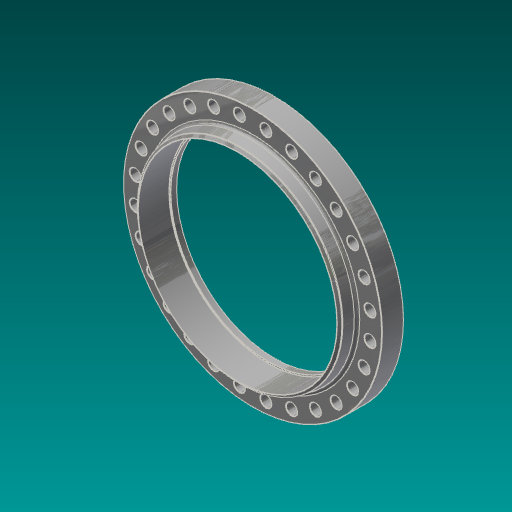
# Autodesk Inventor part: A1-19027-200-03 30in CL300 flange
Saved by Autodesk Inventor 2017.3 (Build 213257000, 257)
## iProperties
Created: 2019-06-26
Part Number: A1-19027-200-03 30in CL300 flange
Material: Steel, Mild
Document SubType Name: Modeling
Designer: Graeme_Van_Dongen
Density: 7.85 g/cm^3
Appearance: Steel
Mass: 267042 g
Surface Area: 19229.6 cm^2
Volume: 34018.1 cm^3
Description: 30" CLASS 300 FFWN FLANGE, A350 LF2, Ø32 1/2" BORE
Author: Graeme_Van_Dongen
Autodesk Inventor part; units mm, degrees
ref_plane "YZ Plane" through (0, 0, 0) normal (1, 0, 0) x (0, 1, 0)
ref_plane "XZ Plane" through (0, 0, 0) normal (0, 1, 0) x (-1, 0, 0)
sketch "Sketch1" plane through (0, 0, 0) normal (0, 0, 1) x (1, 0, 0)
  circle A0 centre (0, 0) radius 546.1
  dimension "d0" = 1092.2
  constraints: 1 centre point, 1 coincident
  measures "d0" diameter of A0
extrude "Extrusion1" add sketch "Sketch1" along normal blind 92.075
sketch "Sketch2" plane through (0, 0, 92.075) normal (0, 0, 1) x (1, 0, 0)
  line L0 (-55.8115, -495.3407) -> (55.8115, 495.3407) construction
  line L1 (0, -764.54) -> (0, 764.54) construction
  point P0 (0, 0)
  point P1 (0, 0)
  dimension "d3" = 996.95
  dimension "d4" = 6.429
  constraints: 2 coincident, 2 end point, 1 midpoint
  measures "d3" distance of L0.start L0.end
  measures "d4" angle of L0 L1
hole "Hole1" at (55.8115, 495.3407, 92.075) direction (0, 0, -1) diameter 47.625 end through all
chamfer "Chamfer1" distance 1.5875 angle 45 2 edges at (55.8115, 519.1532, 92.075) (55.8115, 519.1532, 0)
pattern_circular "Circular Pattern1" count 28 over 360 about axis through (0, 0, -10) along (0, 0, 1) of "Hole1", "Chamfer1"
chamfer "Chamfer2" distance 1.5875 angle 45 2 edges at (-546.1, 0, 92.075) (-546.1, 0, 0)
sketch "Sketch3" plane through (0, 0, 92.075) normal (0, 0, 1) x (1, 0, 0)
  circle A0 centre (0, 0) radius 441.325
  dimension "d21" = 882.65
  constraints: 1 centre point, 1 coincident
  measures "d21" diameter of A0
ref_plane "Work Plane1" through (0, 0, 155.575) normal (0, 0, 1) x (1, 0, 0)
sketch "Sketch4" plane through (0, 0, 155.575) normal (0, 0, 1) x (1, 0, 0)
  circle A0 centre (0, 0) radius 431.8
  dimension "d23" = 863.6
  constraints: 1 centre point, 1 coincident
  measures "d23" diameter of A0
extrude "Extrusion2" add sketch "Sketch4" against normal blind 12.7
loft "Loft1" add profiles "Sketch3" section 1 edges at (-431.8, 0, 142.875)
fillet "Fillet1" radius 12.7 1 edges at (-441.325, 0, 92.075)
sketch "Sketch5" plane through (0, 0, 0) normal (1, 0, 0) x (0, 1, 0)
  line L0 (439.3826, 102.4345) -> (431.8, 142.875) projected
  arc A0 (439.3826, 102.4345) -> (451.8651, 92.075) centre (451.8651, 104.775) ccw projected
  line L1 (431.8, 155.575) -> (431.8, 142.875) construction
  line L2 (0, -30.7975) -> (0, 184.785) projected
  line L3 (0, 0) -> (419.1, 0)
  line L4 (419.1, 0) -> (419.1, 155.575)
  line L5 (420.6875, 155.575) -> (431.8, 147.0481)
  line L6 (431.8, 147.0481) -> (431.8, 142.875)
  line L7 (451.8651, 92.075) -> (451.8651, 155.575)
  line L8 (451.8651, 155.575) -> (0, 155.575)
  dimension "d31" = 863.6
  dimension "d32" = 12.7
  dimension "d33" = 11.1125
  dimension "d37" = 4.1731
  dimension "d49" = 37.5
  constraints: 12 end point, 5 point on line, 2 perpendicular, 1 horizontal, 1 parallel, 1 vertical
  measures "d31" diameter of L6 L2
  measures "d32" distance between parallel lines of L4 L6
  measures "d33" horizontal distance of L5.start L5.end
  measures "d37" distance of L5.end L6.end
  measures "d49" angle of L5 L8
revolve "Revolution1" cut sketch "Sketch5" angle 360 about axis through (0, 0, -10) along (0, 0, 1)
sketch "Sketch6" plane through (0, 0, 0) normal (0, 0, -1) x (-1, 0, 0)
  circle A0 centre (0, 0) radius 412.75
  circle A1 centre (0, 0) radius 419.1 projected
  dimension "d39" = 825.5
  constraints: 1 centre point, 1 coincident
  measures "d39" diameter of A0
extrude "Extrusion3" add sketch "Sketch6" against normal blind 25.4
fillet "Fillet3" radius 0.7937 1 edges at (0, -419.1, 25.4)
chamfer "Chamfer4" distance 0.7937 angle 45 1 edges at (412.75, 0, 25.4)
body "Solid1"
